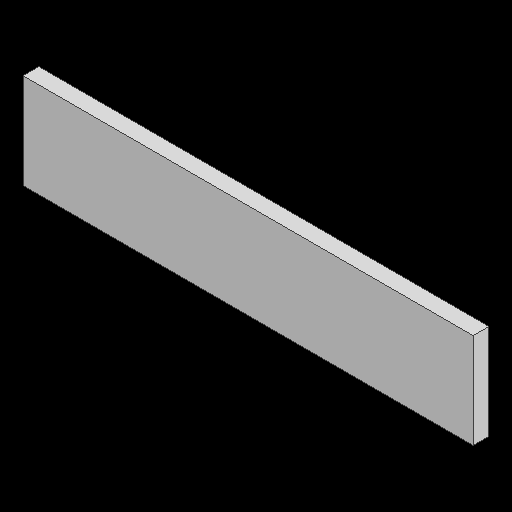
# Autodesk Inventor part: t_pocket
Saved by Autodesk Inventor 2025.1 (Build 291241000, 241)
## iProperties
Created: 2024-08-30
Part Number: t_pocket
Material: 일반
Document SubType Name: Modeling
Designer: ojs08
Density: 1 g/cm^3
Appearance: 기본값
Author: ojs08
Autodesk Inventor part; units mm, degrees
ref_plane "YZ Plane" through (0, 0, 0) normal (1, 0, 0) x (0, 1, 0)
ref_plane "XZ Plane" through (0, 0, 0) normal (0, 1, 0) x (-1, 0, 0)
ref_plane "XY Plane" through (0, 0, 0) normal (0, 0, 1) x (1, 0, 0)
sketch "스케치1" plane through (0, 0, 0) normal (0, 0, 1) x (1, 0, 0)
  line L0 (0, 0) -> (142, 0)
  line L1 (142, 0) -> (142, -30)
  line L2 (142, -30) -> (0, -30)
  line L3 (0, -30) -> (0, 0)
  line L4 (2, -2) -> (28, -2)
  line L5 (28, -2) -> (28, -28)
  line L6 (28, -28) -> (2, -28)
  line L7 (2, -28) -> (2, -2)
  line L8 (56, -2) -> (56, -28)
  line L9 (30, -2) -> (56, -2)
  line L10 (30, -28) -> (30, -2)
  line L11 (56, -28) -> (30, -28)
  line L12 (84, -2) -> (84, -28)
  line L13 (58, -2) -> (84, -2)
  line L14 (58, -28) -> (58, -2)
  line L15 (84, -28) -> (58, -28)
  line L16 (112, -2) -> (112, -28)
  line L17 (86, -2) -> (112, -2)
  line L18 (86, -28) -> (86, -2)
  line L19 (112, -28) -> (86, -28)
  line L20 (140, -2) -> (140, -28)
  line L21 (114, -2) -> (140, -2)
  line L22 (114, -28) -> (114, -2)
  line L23 (140, -28) -> (114, -28)
  dimension "d0" = 142
  dimension "d1" = 30
  dimension "d2" = 2
  dimension "d3" = 2
  dimension "d4" = 26
  dimension "d5" = 26
  dimension "d8" = 28
  constraints: 48 end point, 4 parallel, 3 horizontal, 2 perpendicular, 1 coincident, 32 other
  measures "d0" distance of L1.end L2.end
  measures "d1" distance of L0.end L1.end
  measures "d2" distance between parallel lines of L0 L4
  measures "d3" distance between parallel lines of L3 L7
  measures "d4" distance of L5.end L6.end
  measures "d5" distance of L4.end L5.end
  measures "d8" distance of L4.end L8.start
extrude "돌출1" add sketch "스케치1" along normal blind 4
sketch "스케치2" plane through (0, 0, 4) normal (0, 0, 1) x (1, 0, 0)
  line L0 (0, -30) -> (142, -30) projected
  line L1 (142, -30) -> (142, 0) projected
  line L2 (142, 0) -> (0, 0) projected
  line L3 (0, 0) -> (0, -30) projected
  line L4 (140, -2) -> (140, -28) projected
  line L5 (140, -28) -> (114, -28) projected
  line L6 (114, -28) -> (114, -2) projected
  line L7 (114, -2) -> (140, -2) projected
  line L8 (112, -2) -> (112, -28) projected
  line L9 (112, -28) -> (86, -28) projected
  line L10 (86, -28) -> (86, -2) projected
  line L11 (86, -2) -> (112, -2) projected
  line L12 (84, -2) -> (84, -28) projected
  line L13 (84, -28) -> (58, -28) projected
  line L14 (58, -28) -> (58, -2) projected
  line L15 (58, -2) -> (84, -2) projected
  line L16 (56, -2) -> (56, -28) projected
  line L17 (56, -28) -> (30, -28) projected
  line L18 (30, -28) -> (30, -2) projected
  line L19 (30, -2) -> (56, -2) projected
  line L20 (2, -2) -> (28, -2) projected
  line L21 (28, -2) -> (28, -28) projected
  line L22 (28, -28) -> (2, -28) projected
  line L23 (2, -28) -> (2, -2) projected
extrude "돌출2" add sketch "스케치2" along normal blind 1 contours L3 L2 L1 L0 | L4 L5 L6 L7 | L8 L9 L10 L11 | L12 L13 L14 L15 | L16 L17 L18 L19 | L20 L21 L22 L23
